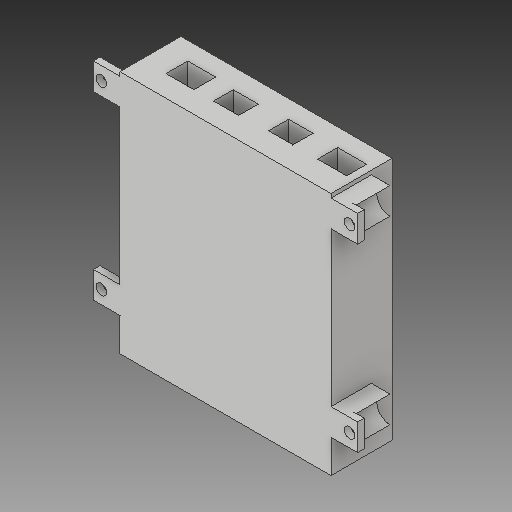
# Autodesk Inventor part: MCM
Saved by Autodesk Inventor 2017 (Build 210142000, 142)
## iProperties
Created: 2022-08-15
Part Number: MCM
Material: Generic
Document SubType Name: Modeling
Designer: JTS
Density: 1 g/cm^3
Appearance: Default
Author: JTS
Autodesk Inventor part; units mm, degrees
ref_plane "YZ Plane" through (0, 0, 0) normal (1, 0, 0) x (0, 1, 0)
ref_plane "XZ Plane" through (0, 0, 0) normal (0, 1, 0) x (-1, 0, 0)
ref_plane "XY Plane" through (0, 0, 0) normal (0, 0, 1) x (1, 0, 0)
sketch "Sketch1" plane through (0, 0, 0) normal (0, 0, 1) x (1, 0, 0)
  line L0 (-79.5, -92) -> (79.5, -92)
  line L1 (79.5, -92) -> (79.5, 92)
  line L2 (79.5, 92) -> (-79.5, 92)
  line L3 (-79.5, 92) -> (-79.5, -92)
  line L4 (-79.5, -92) -> (79.5, 92) construction
  line L5 (79.5, -92) -> (-79.5, 92) construction
  point P0 (0, 0)
  dimension "d0" = 159
  dimension "d1" = 184
  constraints: 12 end point, 2 horizontal, 2 midpoint, 2 vertical
  measures "d0" distance of L1.end L2.end
  measures "d1" distance of L2.end L0.start
extrude "Extrusion1" add sketch "Sketch1" along normal blind 46
sketch "Sketch2" plane through (0, 0, 46) normal (0, 0, 1) x (1, 0, 0)
  line L0 (-79.5, 92) -> (-79.5, -92) projected
  line L1 (79.5, -92) -> (79.5, 92) projected
  line L2 (-79.5, 92) -> (-99.5, 92)
  line L3 (-99.5, 92) -> (-99.5, -92)
  line L4 (-99.5, -92) -> (-79.5, -92)
  line L5 (79.5, -92) -> (99.5, -92)
  line L6 (99.5, -92) -> (99.5, 92)
  line L7 (99.5, 92) -> (79.5, 92)
  point P0 (0, 0)
  dimension "d4" = 20
  constraints: 12 end point, 4 horizontal, 2 vertical, 1 collinear
  measures "d4" distance of L0.start L2.end
extrude "Extrusion2" add sketch "Sketch2" against normal blind 5
sketch "Sketch3" plane through (-79.5, 92, 0) normal (0, 1, 0) x (1, 0, 0)
  line L0 (18.6001, -13.4734) -> (39.6187, -13.4734)
  line L1 (39.6187, -13.4734) -> (39.6187, -29.911)
  line L2 (39.6187, -29.911) -> (18.6001, -29.911)
  line L3 (18.6001, -29.911) -> (18.6001, -13.4734)
  line L4 (54.4394, -15.0902) -> (73.3022, -15.0902)
  line L5 (73.3022, -15.0902) -> (73.3022, -29.911)
  line L6 (73.3022, -29.911) -> (54.4394, -29.911)
  line L7 (54.4394, -29.911) -> (54.4394, -15.0902)
  line L8 (94.5902, -13.4734) -> (112.9141, -13.4734)
  line L9 (112.9141, -13.4734) -> (112.9141, -28.5637)
  line L10 (112.9141, -28.5637) -> (94.5902, -28.5637)
  line L11 (94.5902, -28.5637) -> (94.5902, -13.4734)
  line L12 (131.5074, -13.4734) -> (153.3344, -13.4734)
  line L13 (153.3344, -13.4734) -> (153.3344, -28.5637)
  line L14 (153.3344, -28.5637) -> (131.5074, -28.5637)
  line L15 (131.5074, -28.5637) -> (131.5074, -13.4734)
  point P0 (79.5, 0)
  constraints: 32 end point, 4 point on line
extrude "Extrusion3" cut sketch "Sketch3" against normal blind 25.4
sketch "Sketch4" plane through (0, 0, 46) normal (0, 0, 1) x (1, 0, 0)
  circle A0 centre (-93.5, 79) radius 4
  circle A1 centre (93.5, 79) radius 4
  circle A2 centre (93.5, -57) radius 4
  circle A3 centre (-93.5, -57) radius 4
  line L0 (-99.5, 92) -> (99.5, 92) projected
  line L1 (-99.5, -92) -> (-99.5, 92) projected
  line L2 (99.5, 92) -> (99.5, -92) projected
  line L3 (93.5, 79) -> (-93.5, 79) construction
  line L4 (93.5, 79) -> (93.5, -57) construction
  line L5 (-93.5, -57) -> (-93.5, 79) construction
  line L6 (-99.5, 92) -> (-93.5, 79) construction
  line L7 (93.5, 79) -> (99.5, 92) construction
  line L8 (79.5, 92) -> (79.5, -92) projected
  line L9 (-79.5, -92) -> (-79.5, 92) projected
  line L10 (79.5, 69) -> (99.5, 69)
  line L11 (79.5, -47) -> (99.5, -47)
  line L12 (79.5, -67) -> (99.5, -67)
  line L13 (99.5, -92) -> (79.5, -92)
  line L14 (-79.5, -92) -> (-99.5, -92)
  line L15 (-79.5, -67) -> (-99.5, -67)
  line L16 (-79.5, -47) -> (-99.5, -47)
  line L17 (-79.5, 69) -> (-99.5, 69)
  line L18 (79.5, 89) -> (99.5, 89)
  line L19 (-99.5, 89) -> (-79.5, 89)
  point P0 (0, 0)
  dimension "d9" = 13
  dimension "d10" = 8
  dimension "d11" = 149
  dimension "d12" = 187
  dimension "d13" = 23
  dimension "d14" = 139
  dimension "d15" = 159
  dimension "d22" = 3
  constraints: 30 end point, 16 point on line, 5 horizontal, 4 centre point, 4 collinear, 3 equal radius, 2 equal length, 2 vertical
  measures "d9" distance from line of L0 L3.start
  measures "d10" diameter of A1
  measures "d11" distance from line of L4.end L0
  measures "d12" distance of L3.start L3.end
  measures "d13" distance between parallel lines of L10 L0
  measures "d14" distance between parallel lines of L11 L0
  measures "d15" distance between parallel lines of L0 L12
  measures "d22" distance between parallel lines of L0 L18
extrude "Extrusion4" cut sketch "Sketch4" against normal up to surface (5 mm away) contours A0 | A1 | A2 | A3 | L0 L2 L18 L8 | L0 L9 L19 L1 | L17 L9 L16 L1 | L10 L2 L11 L8 | L15 L9 L14 L1 | L12 L2 L13 L8
sketch "Sketch5" plane through (0, 0, 41) normal (0, 0, -1) x (-1, 0, 0)
  circle A0 centre (-93.5, 79) radius 4 projected
  line L0 (-79.5, 89) -> (-79.5, 69) projected
  line L1 (-99.5, 69) -> (-79.5, 69) projected
  line L2 (-79.5, -47) -> (-99.5, -47) projected
  line L3 (-79.5, -47) -> (-79.5, -67) projected
  line L4 (-99.5, -67) -> (-79.5, -67) projected
  circle A1 centre (-93.5, -57) radius 4 projected
  line L5 (-79.5, 89) -> (-99.5, 89) projected
  line L6 (-93.5, 89) -> (-93.5, 69) construction
  arc A2 (-93.5, 69) -> (-93.5, 89) centre (-93.5, 79) ccw
  line L7 (-93.5, -47) -> (-93.5, -67) construction
  arc A3 (-93.5, -67) -> (-93.5, -47) centre (-93.5, -57) ccw
  point P0 (0, 0)
  constraints: 4 end point, 4 midpoint, 4 point on circle, 4 point on line, 2 centre point, 2 vertical
extrude "Extrusion5" add sketch "Sketch5" along normal blind 25.4 contours L0 L1 A2 L5 | L3 L4 A3 L2
body "Solid1"
